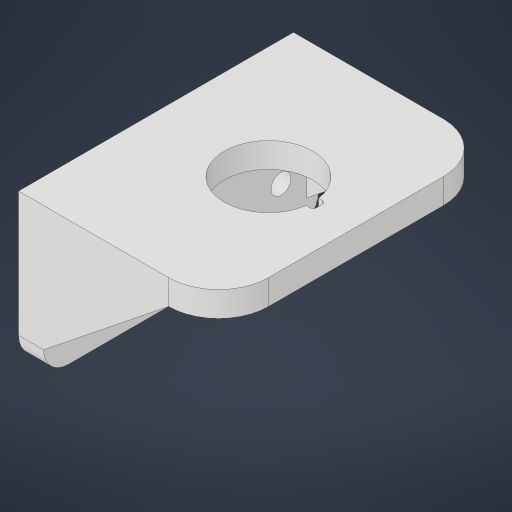
# Autodesk Inventor part: rsl mount
Saved by Autodesk Inventor 2023.4 (Build 274418000, 418)
## iProperties
Created: 2025-02-28
Part Number: rsl mount
Material: ABS Plastic
Document SubType Name: Modeling
Designer: brand
Density: 1.06 g/cm^3
Appearance: Smooth - White
Author: brand
Autodesk Inventor part; units mm, degrees
ref_plane "YZ Plane" through (0, 0, 0) normal (1, 0, 0) x (0, 1, 0)
ref_plane "XZ Plane" through (0, 0, 0) normal (0, 1, 0) x (-1, 0, 0)
ref_plane "XY Plane" through (0, 0, 0) normal (0, 0, 1) x (1, 0, 0)
sketch "Sketch1" plane through (0, 0, 0) normal (0, 0, 1) x (1, 0, 0)
  line L0 (0, 0) -> (50.8, 0)
  line L1 (50.8, 0) -> (50.8, -6.35)
  line L2 (50.8, -6.35) -> (6.35, -6.35)
  line L3 (6.35, -6.35) -> (6.35, -38.1)
  line L4 (6.35, -38.1) -> (0, -38.1)
  line L5 (0, -38.1) -> (0, 0)
  dimension "d0" = 50.8
  dimension "d1" = 38.1
  dimension "d2" = 6.35
  dimension "d3" = 6.35
  constraints: 12 end point, 5 perpendicular, 1 horizontal
  measures "d0" distance of L0.start L0.end
  measures "d1" distance of L4.end L0.start
  measures "d2" distance of L0.end L1.end
  measures "d3" distance of L3.end L4.end
extrude "Extrusion1" add sketch "Sketch1" along normal mid plane 69.85
sketch "Sketch2" plane through (0, 0, 34.925) normal (0, 1, 0) x (1, 0, 0)
  line L0 (0, 69.85) -> (0, 0) construction
  line L1 (50.8, 0) -> (0, 0) construction
  line L2 (50.8, 69.85) -> (50.8, 0) construction
  line L3 (0, 69.85) -> (50.8, 69.85) construction
  circle A0 centre (28.575, 34.925) radius 11.2522
  line L4 (0, 0) -> (0, 69.85) construction
  line L5 (6.35, 69.85) -> (6.35, 0) construction
  line L6 (6.35, 69.85) -> (6.35, 0) construction
  line L7 (6.35, 69.85) -> (6.35, 0) construction
  line L8 (6.35, 69.85) -> (50.8, 69.85) construction
  line L9 (41.525, 36.525) -> (41.525, 33.325)
  line L10 (41.525, 36.525) -> (39.7129, 36.525)
  line L11 (41.525, 33.325) -> (39.7129, 33.325)
  point P0 (0, 34.925)
  point P1 (0, 34.925)
  point P2 (28.575, 69.85)
  point P3 (41.525, 34.925)
  dimension "d6" = 22.5044
  dimension "d16" = 3.2
  dimension "d17" = 12.95
  constraints: 8 end point, 3 midpoint, 2 horizontal, 2 horizontal alignment, 2 point on circle, 1 centre point, 1 perpendicular, 1 vertical, 1 vertical alignment
  measures "d6" diameter of A0
  measures "d16" distance of L9.start L9.end
  measures "d17" distance from line of L9 A0.centre
sketch "Sketch3" plane through (0, -38.1, 34.925) normal (-1, 0, 0) x (0, 0, 1)
  line L0 (0, 0) -> (-69.85, 0) construction
  line L1 (0, 38.1) -> (0, 0) construction
  line L2 (-69.85, 38.1) -> (0, 38.1) construction
  line L3 (-69.85, 0) -> (-69.85, 38.1) construction
  line L4 (-9.525, 25.4) -> (-60.325, 25.4) construction
  line L5 (-60.325, 25.4) -> (-60.325, 12.7) construction
  line L6 (-60.325, 12.7) -> (-9.525, 12.7) construction
  line L7 (-9.525, 12.7) -> (-9.525, 25.4) construction
  line L8 (-9.525, 25.4) -> (-60.325, 12.7) construction
  line L9 (-60.325, 25.4) -> (-9.525, 12.7) construction
  point P0 (-34.925, 38.1)
  point P1 (-34.925, 19.05)
  point P2 (-34.925, 38.1)
  point P3 (0, 19.05)
  dimension "d7" = 50.8
  dimension "d8" = 12.7
  constraints: 12 end point, 4 coincident, 4 midpoint, 2 parallel, 1 horizontal, 1 horizontal alignment, 1 perpendicular, 1 vertical alignment
  measures "d7" distance of L5.end L6.end
  measures "d8" distance of L4.end L5.end
hole "Hole1" at (0, -12.7, -25.4) at (0, -25.4, -25.4) at (0, -25.4, 25.4) at (0, -12.7, 25.4) direction (1, 0, 0) diameter 5.1054 end through all clearance for "Flat Head Machine Screw (82)" size "#10" standard "Ansi Unified Screw Threads"
extrude "Extrusion2" cut sketch "Sketch2" against normal through all
fillet "Fillet1" radius 0.8 2 edges at (41.525, -3.175, -1.6) (41.525, -3.175, 1.6)
fillet "Fillet2" radius 12.7 2 edges at (50.8, -3.175, -34.925) (50.8, -3.175, 34.925)
fillet "Fillet3" radius 6.35 2 edges at (3.175, -38.1, -34.925) (3.175, -38.1, 34.925)
sketch "Sketch5" plane through (0, 0, -34.925) normal (0, 0, -1) x (-1, 0, 0)
  line L0 (0, -31.75) -> (-6.35, -31.75) construction
  line L1 (0, -31.75) -> (0, 0) construction
  line L2 (0, 0) -> (-38.1, 0) construction
  line L3 (-38.1, -6.35) -> (-38.1, 0) construction
  line L4 (-38.1, -6.35) -> (-6.35, -6.35) construction
  line L5 (-6.35, -6.35) -> (-6.35, -31.75) construction
  line L6 (-38.1, -6.35) -> (-6.35, -31.75)
  line L7 (-6.35, -6.35) -> (-6.35, -31.75)
  line L8 (-6.35, -27.9527) -> (-6.35, -22.8473) construction
  line L9 (-6.35, -6.35) -> (-38.1, -6.35)
  line L10 (-17.3228, -6.35) -> (-39.7129, -6.35) construction
  constraints: 6 end point, 2 collinear
extrude "Extrusion3" add sketch "Sketch5" against normal blind 3
mirror "Mirror1" about plane through (0, 0, 0) normal (0, 0, 1) of "Extrusion3"
fillet "Fillet4" radius 6.35 2 edges at (22.225, -6.35, 31.925) (22.225, -6.35, -31.925)
body "Solid1"
